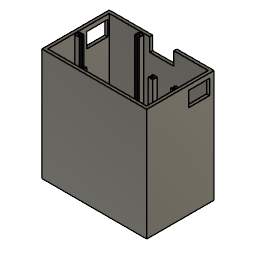
Doos (Autodesk Fusion 360 design; units mm, degrees)
part number: 2026-04-23-13-56-07-142
Autodesk Fusion 360 part; units mm, degrees
sketch "Sketch1" plane through (0, 0, 0) normal (0, 0, 1) x (1, 0, 0)
  line L0 (0, 0) -> (-70, 0)
  line L1 (-70, 0) -> (-70, 45)
  line L2 (-70, 45) -> (0, 45)
  line L3 (0, 45) -> (0, 0)
  constraint horizontal L0
  constraint vertical L1
  constraint horizontal L2
  constraint vertical L3
  constraint coincident L0.start L3.end
extrude "Extrude1" add sketch "Sketch1" along normal blind 75
sketch "Sketch2" plane through (0, 0, 75) normal (0, 0, 1) x (-1, 0, 0)
  line L0 (0, -45) -> (70, -45)
  line L1 (70, -45) -> (70, 0)
  line L2 (70, 0) -> (0, 0)
  line L3 (0, 0) -> (0, -45)
  line L4 (68, -43) -> (2, -43)
  line L5 (2, -43) -> (2, -2)
  line L6 (2, -2) -> (68, -2)
  line L7 (68, -2) -> (68, -43)
  constraint horizontal L4
  constraint vertical L5
  constraint horizontal L6
  constraint vertical L7
extrude "Extrude2" cut sketch "Sketch2" against normal blind 74.8 contours L4 L5 L6 L7
sketch "Sketch3" plane through (0, 0, 0.2) normal (0, 0, 1) x (-1, 0, 0)
  line L0 (68, -2) -> (2, -2)
  line L1 (2, -2) -> (2, -43)
  line L2 (2, -43) -> (68, -43)
  line L3 (68, -43) -> (68, -2)
  line L4 (68, -21) -> (65, -21)
  line L5 (65, -21) -> (65, -20)
  line L6 (65, -20) -> (68, -20)
  line L7 (68, -20) -> (68, -21)
  line L8 (67, -21) -> (68, -21)
  line L9 (68, -21) -> (68, -22)
  line L10 (68, -22) -> (67, -22)
  line L11 (67, -22) -> (67, -21)
  line L12 (68, -23) -> (65, -23)
  line L13 (65, -23) -> (65, -22)
  line L14 (65, -22) -> (68, -22)
  line L15 (68, -22) -> (68, -23)
  line L16 (19, -22) -> (16, -22)
  line L17 (16, -22) -> (16, -23)
  line L18 (16, -23) -> (19, -23)
  line L19 (19, -23) -> (19, -22)
  line L20 (17, -22) -> (16, -22)
  line L21 (16, -22) -> (16, -21)
  line L22 (16, -21) -> (17, -21)
  line L23 (17, -21) -> (17, -22)
  line L24 (16, -21) -> (19, -21)
  line L25 (19, -21) -> (19, -20)
  line L26 (19, -20) -> (16, -20)
  line L27 (16, -20) -> (16, -21)
  constraint horizontal L4
  constraint vertical L5
  constraint horizontal L6
  constraint vertical L7
  constraint horizontal L8
  constraint vertical L9
  constraint horizontal L10
  constraint vertical L11
  constraint coincident L3 L9.end
  constraint coincident L4 L8.start
  constraint horizontal L12
  constraint vertical L13
  constraint horizontal L14
  constraint vertical L15
  constraint coincident L3 L12.start
  constraint horizontal L16
  constraint vertical L17
  constraint horizontal L18
  constraint vertical L19
  constraint horizontal L20
  constraint vertical L21
  constraint horizontal L22
  constraint vertical L23
  constraint horizontal L24
  constraint vertical L25
  constraint horizontal L26
  constraint vertical L27
extrude "Extrude3" add sketch "Sketch3" along normal blind 74 contours L3 L4 L5 L6 L7 L8 | L3 L4 L8 L9 L10 L11 L14 | L3 L10 L12 L13 L14 L15 | L16 L17 L18 L19 L20 | L16 L20 L21 L22 L23 L24 | L22 L24 L25 L26 L27
sketch "Sketch4" plane through (-68, 0, 0) normal (1, 0, 0) x (0, 1, 0)
  line L0 (23, 74.2) -> (23, 0.2)
  line L1 (23, 0.2) -> (43, 0.2)
  line L2 (43, 0.2) -> (43, 75)
  line L3 (43, 75) -> (2, 75)
  line L4 (2, 75) -> (2, 0.2)
  line L5 (2, 0.2) -> (20, 0.2)
  line L6 (20, 0.2) -> (20, 74.2)
  line L7 (20, 74.2) -> (23, 74.2)
  line L8 (28, 72) -> (42, 72)
  line L9 (42, 72) -> (42, 62)
  line L10 (42, 62) -> (28, 62)
  line L11 (28, 62) -> (28, 72)
  constraint horizontal L8
  constraint vertical L9
  constraint horizontal L10
  constraint vertical L11
extrude "Extrude4" cut sketch "Sketch4" against normal blind 8 contours L8 L9 L10 L11
sketch "Sketch5" plane through (0, 0, 0) normal (1, 0, 0) x (0, 1, 0)
  line L0 (0, 0) -> (45, 0)
  line L1 (45, 0) -> (45, 75)
  line L2 (45, 75) -> (0, 75)
  line L3 (0, 75) -> (0, 0)
  line L4 (42, 72) -> (28, 72)
  line L5 (28, 72) -> (28, 62)
  line L6 (28, 62) -> (42, 62)
  line L7 (42, 62) -> (42, 72)
  constraint horizontal L4
  constraint vertical L5
  constraint horizontal L6
  constraint vertical L7
extrude "Extrude5" cut sketch "Sketch5" against normal blind 9 contours L4 L5 L6 L7
sketch "Sketch6" plane through (0, 43, 0) normal (0, -1, 0) x (1, 0, 0)
  line L0 (-2, 75) -> (-68, 75)
  line L1 (-68, 75) -> (-68, 0.2)
  line L2 (-68, 0.2) -> (-2, 0.2)
  line L3 (-2, 0.2) -> (-2, 75)
  line L4 (-41, 75) -> (-25, 75)
  line L5 (-25, 75) -> (-25, 66)
  line L6 (-25, 66) -> (-41, 66)
  line L7 (-41, 66) -> (-41, 75)
  constraint horizontal L4
  constraint vertical L5
  constraint horizontal L6
  constraint vertical L7
  constraint coincident L0 L4.end
extrude "Extrude6" cut sketch "Sketch6" against normal blind 8 contours L0 L4 L5 L6 L7
sketch "Sketch7" plane through (0, 0, 0) normal (0, 0, -1) x (1, 0, 0)
  line L0 (-70, -45) -> (0, -45)
  line L1 (0, -45) -> (0, 0)
  line L2 (0, 0) -> (-70, 0)
  line L3 (-70, 0) -> (-70, -45)
  line L4 (-64, -5) -> (-60, -5)
  line L5 (-60, -5) -> (-60, -7)
  line L6 (-60, -7) -> (-64, -7)
  line L7 (-64, -7) -> (-64, -5)
  line L8 (-64, -40) -> (-60, -40)
  line L9 (-60, -40) -> (-60, -38)
  line L10 (-60, -38) -> (-64, -38)
  line L11 (-64, -38) -> (-64, -40)
  line L12 (-6, -5) -> (-10, -5)
  line L13 (-10, -5) -> (-10, -7)
  line L14 (-10, -7) -> (-6, -7)
  line L15 (-6, -7) -> (-6, -5)
  line L16 (-6, -38) -> (-10, -38)
  line L17 (-10, -38) -> (-10, -40)
  line L18 (-10, -40) -> (-6, -40)
  line L19 (-6, -40) -> (-6, -38)
  constraint horizontal L4
  constraint vertical L5
  constraint horizontal L6
  constraint vertical L7
  constraint horizontal L8
  constraint vertical L9
  constraint horizontal L10
  constraint vertical L11
  constraint horizontal L12
  constraint vertical L13
  constraint horizontal L14
  constraint vertical L15
  constraint horizontal L16
  constraint vertical L17
  constraint horizontal L18
  constraint vertical L19
extrude "Extrude7" add sketch "Sketch7" along normal blind 4 contours L4 L5 L6 L7 | L8 L9 L10 L11 | L12 L13 L14 L15 | L16 L17 L18 L19
sketch "Sketch8" plane through (0, 7, 0) normal (0, 1, 0) x (-1, 0, 0)
  line L0 (64, 0) -> (60, 0)
  line L1 (60, 0) -> (60, -4)
  line L2 (60, -4) -> (64, -4)
  line L3 (64, -4) -> (64, 0)
  line L4 (64, -4) -> (60, -4)
  line L5 (60, -4) -> (60, -2)
  line L6 (60, -2) -> (64, -2)
  line L7 (64, -2) -> (64, -4)
  constraint horizontal L4
  constraint vertical L5
  constraint horizontal L6
  constraint vertical L7
  constraint midpoint L1 L5.end
  constraint coincident L2.end L3.start
extrude "Extrude8" add sketch "Sketch8" along normal blind 31 contours L1 L2 L3 L4 L5 L6 L7
sketch "Sketch9" plane through (0, 7, 0) normal (0, 1, 0) x (-1, 0, 0)
  line L0 (10, 0) -> (6, 0)
  line L1 (6, 0) -> (6, -4)
  line L2 (6, -4) -> (10, -4)
  line L3 (10, -4) -> (10, 0)
  line L4 (10, -4) -> (6, -4)
  line L5 (6, -4) -> (6, -2)
  line L6 (6, -2) -> (10, -2)
  line L7 (10, -2) -> (10, -4)
  constraint horizontal L4
  constraint vertical L5
  constraint horizontal L6
  constraint vertical L7
  constraint midpoint L1 L5.end
  constraint coincident L2.end L3.start
extrude "Extrude9" add sketch "Sketch9" along normal blind 31 contours L1 L2 L3 L4 L5 L6 L7
sketch "Sketch10" plane through (0, 0, 0.2) normal (0, 0, 1) x (-1, 0, 0)
  line L0 (68, -23) -> (65, -23)
  line L1 (65, -23) -> (65, -22)
  line L2 (65, -22) -> (67, -22)
  line L3 (67, -22) -> (67, -21)
  line L4 (67, -21) -> (65, -21)
  line L5 (65, -21) -> (65, -20)
  line L6 (65, -20) -> (68, -20)
  line L7 (68, -20) -> (68, -2)
  line L8 (68, -2) -> (2, -2)
  line L9 (2, -2) -> (2, -43)
  line L10 (2, -43) -> (68, -43)
  line L11 (68, -43) -> (68, -23)
  line L12 (17, -21) -> (17, -22)
  line L13 (17, -22) -> (19, -22)
  line L14 (19, -22) -> (19, -23)
  line L15 (19, -23) -> (16, -23)
  line L16 (16, -23) -> (16, -20)
  line L17 (16, -20) -> (19, -20)
  line L18 (19, -20) -> (19, -21)
  line L19 (19, -21) -> (17, -21)
  line L20 (2, -21) -> (3, -21)
  line L21 (3, -21) -> (3, -24)
  line L22 (3, -24) -> (2, -24)
  line L23 (2, -24) -> (2, -21)
  line L24 (3, -24) -> (5, -24)
  line L25 (5, -24) -> (5, -23)
  line L26 (5, -23) -> (3, -23)
  line L27 (3, -23) -> (3, -24)
  line L28 (3, -21) -> (5, -21)
  line L29 (5, -21) -> (5, -22)
  line L30 (5, -22) -> (3, -22)
  line L31 (3, -22) -> (3, -21)
  line L32 (45, -43) -> (46, -43)
  line L33 (46, -43) -> (46, -40)
  line L34 (46, -40) -> (45, -40)
  line L35 (45, -40) -> (45, -43)
  line L36 (46, -43) -> (47, -43)
  line L37 (47, -43) -> (47, -42)
  line L38 (47, -42) -> (46, -42)
  line L39 (46, -42) -> (46, -43)
  line L40 (48, -43) -> (47, -43)
  line L41 (47, -43) -> (47, -40)
  line L42 (47, -40) -> (48, -40)
  line L43 (48, -40) -> (48, -43)
  line L44 (45, -2) -> (46, -2)
  line L45 (46, -2) -> (46, -5)
  line L46 (46, -5) -> (45, -5)
  line L47 (45, -5) -> (45, -2)
  line L48 (46, -2) -> (47, -2)
  line L49 (47, -2) -> (47, -3)
  line L50 (47, -3) -> (46, -3)
  line L51 (46, -3) -> (46, -2)
  line L52 (47, -2) -> (48, -2)
  line L53 (48, -2) -> (48, -5)
  line L54 (48, -5) -> (47, -5)
  line L55 (47, -5) -> (47, -2)
  constraint horizontal L20
  constraint vertical L21
  constraint horizontal L22
  constraint vertical L23
  constraint coincident L9 L20.start
  constraint horizontal L24
  constraint vertical L25
  constraint horizontal L26
  constraint vertical L27
  constraint horizontal L28
  constraint vertical L29
  constraint horizontal L30
  constraint vertical L31
  constraint horizontal L32
  constraint vertical L33
  constraint horizontal L34
  constraint vertical L35
  constraint coincident L10 L32.start
  constraint horizontal L36
  constraint vertical L37
  constraint horizontal L38
  constraint vertical L39
  constraint horizontal L40
  constraint vertical L41
  constraint horizontal L42
  constraint vertical L43
  constraint coincident L10 L40.start
  constraint horizontal L44
  constraint vertical L45
  constraint horizontal L46
  constraint vertical L47
  constraint coincident L8 L44.start
  constraint horizontal L48
  constraint vertical L49
  constraint horizontal L50
  constraint vertical L51
  constraint horizontal L52
  constraint vertical L53
  constraint horizontal L54
  constraint vertical L55
extrude "Extrude10" add sketch "Sketch10" along normal blind 74 contours L10 L37 L40 L41 L42 L43 | L10 L33 L36 L37 L38 L39 L41 | L10 L32 L33 L34 L35 L39 | L9 L20 L21 L22 L23 L27 L31 | L21 L24 L25 L26 L27 | L8 L49 L52 L53 L54 L55 | L21 L28 L29 L30 L31 | L8 L45 L48 L49 L50 L51 L55 | L8 L44 L45 L46 L47 L51
sketch "Sketch11" plane through (0, 45, 0) normal (0, 1, 0) x (-1, 0, 0)
  line L0 (25, 66) -> (25, 75)
  line L1 (41, 75) -> (41, 66)
  line L2 (41, 66) -> (25, 66)
  line L3 (0, 0) -> (70, 0)
  line L4 (70, 0) -> (70, 75)
  line L5 (25, 75) -> (0, 75)
  line L6 (0, 75) -> (0, 0)
  line L7 (25, 66) -> (21, 66)
  line L8 (21, 66) -> (21, 72)
  line L9 (21, 72) -> (25, 72)
  line L10 (25, 72) -> (25, 66)
  line L11 (70, 75) -> (41, 75)
  constraint horizontal L7
  constraint vertical L8
  constraint horizontal L9
  constraint vertical L10
  constraint coincident L0.start L2.end
extrude "Extrude11" cut sketch "Sketch11" against normal blind 4 contours L0 L7 L8 L9 L10
extrude "Extrude12" add sketch "Sketch11" against normal blind 2 contours L0 L7 L8 L9 L10
